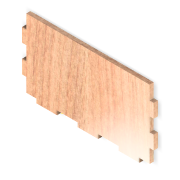
# Autodesk Inventor part: zijkant2 electronica
Saved by Autodesk Inventor 2020.3 (Build 243373000, 373)
## iProperties
Created: 2020-10-19
Part Number: zijkant2 electronica
Material: Wood (Birch)
Document SubType Name: Sheet Metal
Designer: Svend
Density: 0.55 g/cm^3
Sheet Metal Rule: Default_mm
Appearance: Birch - Natural Polished
Author: Svend
Autodesk Inventor part; units mm, degrees
ref_plane "YZ Plane" through (0, 0, 0) normal (1, 0, 0) x (0, 1, 0)
ref_plane "XZ Plane" through (0, 0, 0) normal (0, 1, 0) x (-1, 0, 0)
ref_plane "XY Plane" through (0, 0, 0) normal (0, 0, 1) x (1, 0, 0)
ref_plane "Work Plane1" through (0, 0, 0) normal (0, 0, 1) x (1, 0, 0)
sketch "Sketch1" plane through (0, 0, 0) normal (0, 0, 1) x (1, 0, 0)
  line L0 (0, 0) -> (30, 0)
  line L1 (0, 0) -> (0, -6)
  line L2 (30, -6) -> (0, -6)
  line L3 (30, 0) -> (30, -6)
  line L4 (60, 0) -> (90, 0)
  line L5 (60, 0) -> (60, -6)
  line L6 (90, -6) -> (60, -6)
  line L7 (90, 0) -> (90, -6)
  line L8 (120, 0) -> (150, 0)
  line L9 (120, 0) -> (120, -6)
  line L10 (150, -6) -> (120, -6)
  line L11 (150, 0) -> (150, -6)
  line L12 (30, 0) -> (60, 0)
  line L13 (90, 0) -> (120, 0)
  line L14 (150, 0) -> (164.8734, 0)
  line L15 (0, 0) -> (-14.8734, 0)
  line L16 (-20.8734, -6) -> (0, -6)
  line L17 (150, -6) -> (170.8734, -6)
  line L18 (0, 0) -> (0, -6)
  line L19 (30, -6) -> (0, -6)
  line L20 (30, -6) -> (30, 0)
  line L21 (60, 0) -> (60, -6)
  line L22 (90, -6) -> (60, -6)
  line L23 (90, -6) -> (90, 0)
  line L24 (120, 0) -> (120, -6)
  line L25 (120, -6) -> (150, -6)
  line L26 (150, 0) -> (150, -6)
  line L27 (164.8734, 0) -> (164.8734, 100)
  line L28 (-14.8734, 0) -> (-14.8734, 100)
  line L29 (-14.8734, 100) -> (164.8734, 100)
  line L30 (164.8734, 20) -> (170.8734, 20)
  line L31 (170.8734, 20) -> (170.8734, 40)
  line L32 (170.8734, 40) -> (164.8734, 40)
  line L33 (164.8734, 40) -> (164.8734, 20)
  line L34 (164.8734, 60) -> (170.8734, 60)
  line L35 (170.8734, 60) -> (170.8734, 80)
  line L36 (170.8734, 80) -> (164.8734, 80)
  line L37 (164.8734, 80) -> (164.8734, 60)
  line L38 (-14.8734, 80) -> (-20.8734, 80)
  line L39 (-20.8734, 80) -> (-20.8734, 60)
  line L40 (-20.8734, 60) -> (-14.8734, 60)
  line L41 (-14.8734, 60) -> (-14.8734, 80)
  line L42 (-14.8734, 20) -> (-20.8734, 20)
  line L43 (-20.8734, 20) -> (-20.8734, 40)
  line L44 (-20.8734, 40) -> (-14.8734, 40)
  line L45 (-14.8734, 40) -> (-14.8734, 20)
  dimension "d0" = 6
  dimension "d1" = 6
  dimension "d2" = 100
  dimension "d3" = 100
  dimension "d5" = 20
  dimension "d6" = 20
  dimension "d7" = 20
  dimension "d8" = 6
  measures "d0" horizontal distance of L14.end L17.end
  measures "d1" horizontal distance of L15.end L16.start
  measures "d2" distance of L14.end L27.end
  measures "d3" distance of L15.end L28.end
  measures "d5" distance of L38.end L39.end
  measures "d6" distance from line of L28.end L38
  measures "d7" distance between parallel lines of L44 L40
  measures "d8" distance between parallel lines of L43 L28
extrude "Plate1" add sketch "Sketch1" along normal blind 6
equation "\"d6\" = d5"
equation "\"d7\" = d5"
equation "\"d4\" = Thickness"
equation "\"BendRadius\" = Thickness"
equation "\"BendReliefWidth\" = Thickness"
equation "\"BendReliefDepth\" = 0.5 * Thickness"
equation "\"CornerReliefSize\" = 4 * Thickness"
equation "\"MinimumRemnant\" = 2 * Thickness"
equation "\"TransitionRadius\" = BendRadius"
equation "\"JacobiRadiusSize\" = BendRadius"
equation "\"GapSize\" = Thickness"
equation "\"Thickness\" = 6"
body "Solid1"
